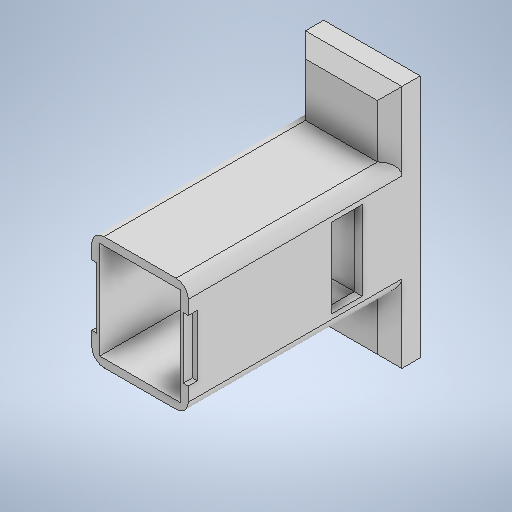
# Autodesk Inventor part: VL53L0X_case
Saved by Autodesk Inventor 2025.3 (Build 293356000, 356)
## iProperties
Created: 2025-11-14
Part Number: VL53L0X_case
Material: Generic
Document SubType Name: Modeling
Designer: woyao
Density: 1 g/cm^3
Appearance: Default
Author: woyao
Autodesk Inventor part; units mm, degrees
ref_plane "YZ Plane" through (0, 0, 0) normal (1, 0, 0) x (0, 1, 0)
ref_plane "XZ Plane" through (0, 0, 0) normal (0, 1, 0) x (-1, 0, 0)
sketch "Sketch1" plane through (0, 0, 0) normal (0, 0, 1) x (1, 0, 0)
  point P0 (0, 0)
sketch "Sketch2" plane through (0, 0, 0) normal (0, 0, 1) x (1, 0, 0)
  line L0 (0, 0) -> (13.2, 0)
  line L1 (13.2, 0) -> (13.2, 16)
  line L2 (13.2, 16) -> (0, 16)
  line L3 (0, 16) -> (0, 0)
  line L4 (14.5, 17.3) -> (14.5, -1.3)
  line L5 (14.5, -1.3) -> (-1.3, -1.3)
  line L6 (-1.3, -1.3) -> (-1.3, 17.3)
  line L7 (-1.3, 17.3) -> (14.5, 17.3)
  dimension "d0" = 13.2
  dimension "d1" = 16
  dimension "d2" = 1.3
  constraints: 16 end point, 4 parallel, 2 perpendicular, 1 horizontal, 3 other
  measures "d0" distance of L1.end L2.end
  measures "d1" distance of L0.end L1.end
  measures "d2" distance between parallel lines of L1 L4
extrude "Extrusion1" add sketch "Sketch2" along normal blind 30
sketch "Sketch3" plane through (0, 0, 0) normal (0, 0, -1) x (-1, 0, 0)
  line L0 (-14.5, -1.3) -> (-14.5, 17.3) projected
  line L1 (1.3, 17.3) -> (1.3, -1.3) projected
  line L2 (-14.5, 17.3) -> (1.3, 17.3) projected
  line L3 (1.3, -1.3) -> (-14.5, -1.3) projected
  line L4 (1.3, 17.3) -> (-14.5, 17.3)
  line L5 (-14.5, 17.3) -> (-14.5, 25.3)
  line L6 (-14.5, 25.3) -> (1.3, 25.3)
  line L7 (1.3, 25.3) -> (1.3, 17.3)
  line L8 (1.3, -1.3) -> (-14.5, -1.3)
  line L9 (-14.5, -1.3) -> (-14.5, -9.3)
  line L10 (-14.5, -9.3) -> (1.3, -9.3)
  line L11 (1.3, -9.3) -> (1.3, -1.3)
  point P0 (0, 0)
  dimension "d27" = 8
  dimension "d28" = 8
  constraints: 16 end point, 4 parallel, 2 horizontal, 2 perpendicular, 1 point on line
  measures "d27" distance of L4.end L5.end
  measures "d28" distance of L8.end L9.end
extrude "Extrusion2" add sketch "Sketch3" along normal blind 3 contours L0 L2 L1 L3
sketch "Sketch5" plane through (14.5, -1.3, 30) normal (1, 0, 0) x (0, 0, -1)
  line L0 (28.5, 2.8) -> (23.5, 2.8)
  line L1 (23.5, 2.8) -> (23.5, 15.8)
  line L2 (23.5, 15.8) -> (28.5, 15.8)
  line L3 (28.5, 15.8) -> (28.5, 2.8)
  line L4 (33, 0) -> (0, 0) projected
  line L5 (33, 18.6) -> (33, 0) projected
  point P0 (30, 1.3)
  point P1 (30, 0)
  dimension "d14" = 13
  dimension "d15" = 5
  dimension "d16" = 2.8
  dimension "d17" = 4.5
  constraints: 8 end point, 2 parallel, 1 horizontal, 1 perpendicular
  measures "d14" distance of L0.end L1.end
  measures "d15" distance of L0.start L0.end
  measures "d16" distance between parallel lines of L0 L4
  measures "d17" distance between parallel lines of L5 L3
extrude "Extrusion4" cut sketch "Sketch5" against normal blind 1.3
sketch "Sketch6" plane through (-1.3, -1.3, 30) normal (-1, 0, 0) x (0, 0, 1)
  line L0 (0, 17.3) -> (0, 1.3) projected
  line L1 (0, 14.3) -> (-1.5, 14.3)
  line L2 (-1.5, 14.3) -> (-1.5, 4.3)
  line L3 (-1.5, 4.3) -> (0, 4.3)
  line L4 (0, 4.3) -> (0, 14.3)
  line L5 (0, 18.6) -> (-33, 18.6) projected
  point P0 (-30, 1.3)
  point P1 (0, 4.3)
  dimension "d20" = 10
  dimension "d21" = 1.5
  dimension "d30" = 4.3
  constraints: 8 end point, 2 parallel, 1 horizontal, 1 perpendicular, 1 point on line
  measures "d20" distance of L1.end L2.end
  measures "d21" distance of L2.end L3.end
  measures "d30" distance between parallel lines of L1 L5
sketch "Sketch7" plane through (14.5, -1.3, 30) normal (1, 0, 0) x (0, 0, -1)
  line L0 (1.5, 14.3) -> (1.5, 4.3) projected
  line L1 (0, 14.3) -> (1.5, 14.3) projected
  line L2 (1.5, 4.3) -> (0, 4.3) projected
  line L3 (0, 14.3) -> (0, 4.3)
  line L4 (0, 18.6) -> (0, 0) projected
  point P0 (30, 1.3)
  point P1 (0, 14.3)
  constraints: 2 end point, 1 collinear
ref_plane "Work Plane1" through (6.6, -1.3, -3) normal (1, 0, 0) x (0, 0, -1)
extrude "Extrusion7" cut sketch "Sketch7" against normal blind 0.8
extrude "Extrusion8" cut sketch "Sketch6" against normal blind 0.8
sketch "Sketch8" plane through (0, 0, -3) normal (0, 0, -1) x (-1, 0, 0)
  line L0 (-14.5, 28) -> (1.3, 28)
  line L1 (1.3, 28) -> (1.3, -12)
  line L2 (1.3, -12) -> (-14.5, -12)
  line L3 (-14.5, -12) -> (-14.5, 28)
  line L4 (1.3, 17.3) -> (-14.5, 17.3) projected
  line L5 (-14.5, -1.3) -> (1.3, -1.3) projected
  line L6 (-14.5, 17.3) -> (1.3, 17.3) projected
  line L7 (-14.5, 17.3) -> (-14.5, -1.3) projected
  line L8 (1.3, -1.3) -> (1.3, 17.3) projected
  line L9 (-14.5, 8) -> (1.3, 8) construction
  point P0 (0, 0)
  dimension "d39" = 40
  dimension "d40" = 20
  constraints: 10 end point, 2 collinear, 2 midpoint, 1 parallel
  measures "d39" distance between parallel lines of L2 L0
  measures "d40" distance between parallel lines of L0 L9
extrude "Extrusion9" add sketch "Sketch8" along normal blind 5
fillet "Fillet2" radius 2 4 edges at (14.5, 17.3, 13.5) (-1.3, 17.3, 13.5) (14.5, -1.3, 13.5) (-1.3, -1.3, 13.5)
chamfer "Chamfer1" distance 2 angle 45 6 edges at (-1.3, 16.3, -3) (14.5, 16.3, -3) (-1.3, -0.3, -3) (14.5, -0.3, -3) (6.6, -12, -3) (6.6, 28, -3)
body "Solid1"
